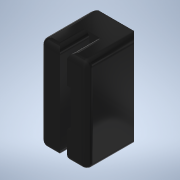
# Autodesk Inventor part: SP45V1 Plastico Roldana
Saved by Autodesk Inventor 2021.2 (Build 252289000, 289)
## iProperties
Created: 2026-09-01
Part Number: SP45V1 Plastico Roldana
Material: ABS Plastic
Document SubType Name: Modeling
Designer: nelso
Density: 1.06 g/cm^3
Appearance: Smooth - Black
Author: nelso
Autodesk Inventor part; units mm, degrees
ref_plane "YZ Plane" through (0, 0, 0) normal (1, 0, 0) x (0, 1, 0)
ref_plane "XZ Plane" through (0, 0, 0) normal (0, 1, 0) x (-1, 0, 0)
sketch "Sketch1" plane through (0, 0, 0) normal (0, 1, 0) x (-1, 0, 0)
  line L0 (-20, 40) -> (20, 40)
  line L1 (20, 40) -> (20, -40)
  line L2 (20, -40) -> (-20, -40)
  line L3 (-20, -40) -> (-20, 40)
  line L4 (-20, 40) -> (20, -40) construction
  line L5 (20, 40) -> (-20, -40) construction
  point P0 (0, 0)
  dimension "d0" = 40
  dimension "d1" = 80
  constraints: 12 end point, 2 midpoint, 2 parallel, 1 horizontal, 1 perpendicular
  measures "d0" distance of L1.end L2.end
  measures "d1" distance of L0.end L1.end
extrude "Extrusion1" add sketch "Sketch1" along normal mid plane 45
sketch "Sketch2" plane through (0, -22.5, 0) normal (0, -1, 0) x (1, 0, 0)
  line L0 (20, -40) -> (-20, -40) projected
  line L1 (3, 40) -> (-3, 40)
  line L2 (-3, 40) -> (-3, -40)
  line L3 (-3, -40) -> (3, -40)
  line L4 (3, -40) -> (3, 40)
  line L5 (3, 40) -> (-3, -40) construction
  line L6 (-3, 40) -> (3, -40) construction
  point P0 (0, 0)
  dimension "d4" = 6
  constraints: 12 end point, 2 midpoint, 2 parallel, 1 horizontal, 1 perpendicular, 1 point on line
  measures "d4" distance of L3.end L2.end
extrude "Extrusion2" cut sketch "Sketch2" against normal blind 25
chamfer "Chamfer1" distance 5 angle 45 2 edges at (20, 22.5, 0) (-20, 22.5, 0)
chamfer "Chamfer2" distance 0.3 angle 45 2 edges at (0, 22.5, 40) (0, 22.5, -40)
fillet "Fillet1" radius 5 14 edges at (20, -2.5, 40) (-20, -2.5, 40) (20, -2.5, -40) (-20, -2.5, -40) (3, -10, -40) (-3, -10, -40) (-3, -10, 40) (3, -10, 40) (-20, -22.5, 0) (-11.5, -22.5, 40) (-11.5, -22.5, -40) (11.5, -22.5, -40) (20, -22.5, 0) (11.5, -22.5, 40)
sketch "Sketch5" plane through (3, -22.5, -35) normal (-1, 0, 0) x (0, 0, 1)
  line L0 (70, 0) -> (0, 0) projected
  line L1 (35, 0) -> (19, 0)
  line L2 (70, 25) -> (0, 25) projected
  line L3 (19, 0) -> (19, 25)
  line L4 (19, 25) -> (51, 25)
  line L5 (51, 25) -> (51, 0)
  line L6 (51, 0) -> (19, 0)
  point P0 (51, 0)
  dimension "d31" = 16
  dimension "d32" = 32
  constraints: 10 end point, 2 parallel, 2 point on line, 1 midpoint, 1 perpendicular, 1 vertical
  measures "d31" distance of L1.start L1.end
  measures "d32" distance of L3.end L4.end
extrude "Extrusion4" cut sketch "Sketch5" against normal blind 3
sketch "Sketch6" plane through (6, -22.5, -35) normal (-1, 0, 0) x (0, 0, 1)
  line L0 (19, 25) -> (51, 25) projected
  line L1 (19, 0) -> (19, 25) projected
  line L2 (51, 0) -> (19, 0) projected
  line L3 (51, 25) -> (51, 0) projected
  line L4 (19, 25) -> (51, 25) projected
  line L5 (35, 25) -> (35, 18)
  line L6 (35, 18) -> (25, 18)
  point P0 (35, 22.5)
  point P1 (45, 18)
  dimension "d35" = 7
  dimension "d36" = 10
  constraints: 4 end point, 1 coincident, 1 midpoint, 1 perpendicular, 1 symmetric about line, 1 vertical
  measures "d35" distance of L5.start L5.end
  measures "d36" distance of L5.end L6.end
hole "Hole2" at (6, -4.5, -10) at (6, -4.5, 10) direction (1, 0, 0) diameter 3.6 depth 8 clearance for "Countersunk Flat Head Screw ISO 2009/7046" size "M3" standard "ISO"
ref_plane "Work Plane1" through (11.5, -22.5, 35) normal (-1, 0, 0) x (0, 0, 1)
sketch "Sketch7" plane through (11.5, -22.5, 35) normal (-1, 0, 0) x (0, 0, 1)
  line L0 (-25, 14.4204) -> (-28.1, 16.2102)
  line L1 (-28.1, 16.2102) -> (-28.1, 19.7898)
  line L2 (-28.1, 19.7898) -> (-25, 21.5796)
  line L3 (-25, 21.5796) -> (-21.9, 19.7898)
  line L4 (-21.9, 19.7898) -> (-21.9, 16.2102)
  line L5 (-21.9, 16.2102) -> (-25, 14.4204)
  line L6 (-45, 14.4204) -> (-48.1, 16.2102)
  line L7 (-48.1, 16.2102) -> (-48.1, 19.7898)
  line L8 (-48.1, 19.7898) -> (-45, 21.5796)
  line L9 (-45, 21.5796) -> (-41.9, 19.7898)
  line L10 (-41.9, 19.7898) -> (-41.9, 16.2102)
  line L11 (-41.9, 16.2102) -> (-45, 14.4204)
  line L12 (-21.9, 16.2102) -> (-21.9, 14.4204)
  line L13 (-21.9, 14.4204) -> (-28.1, 14.4204)
  line L14 (-28.1, 14.4204) -> (-28.1, 16.2102)
  line L15 (-41.9, 16.2102) -> (-41.9, 14.4204)
  line L16 (-41.9, 14.4204) -> (-48.1, 14.4204)
  line L17 (-48.1, 14.4204) -> (-48.1, 16.2102)
  point P0 (-35, 22.5)
  point P1 (-25, 18)
  point P2 (-45, 18)
  point P3 (-25, 18)
  point P4 (-45, 18)
  dimension "d52" = 6.2
  dimension "d53" = 6.2
  constraints: 36 end point, 3 perpendicular, 2 coincident, 2 point on line, 1 parallel, 1 vertical, 26 other
  measures "d52" distance between parallel lines of L1 L4
  measures "d53" distance between parallel lines of L7 L10
extrude "Extrusion5" cut sketch "Sketch7" along normal blind 3.6
sketch "Sketch8" plane through (-20, -17.5, -35) normal (-1, 0, 0) x (0, 0, 1)
  circle A0 centre (25, 13) radius 1.8 projected
  circle A1 centre (45, 13) radius 1.8 projected
  line L0 (19, 20) -> (51, 20) projected
  line L1 (19, -5) -> (19, 20) projected
  line L2 (51, -5) -> (19, -5) projected
  line L3 (51, 20) -> (51, -5) projected
  circle A2 centre (25, 13) radius 3.5
  circle A3 centre (45, 13) radius 3.5
  point P0 (35, 17.5)
  dimension "d48" = 7
  dimension "d49" = 7
  constraints: 2 centre point, 2 coincident
  measures "d48" diameter of A2
  measures "d49" diameter of A3
extrude "Extrusion6" cut sketch "Sketch8" against normal up to surface (23 mm away) contours A0 | A1 | A2 | A3
body "Solid1"
